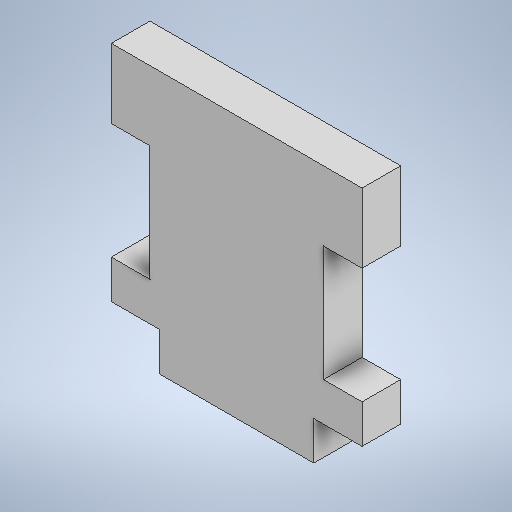
# Autodesk Inventor part: Manija3
Saved by Autodesk Inventor 2025 (Build 290162000, 162)
## iProperties
Created: 2024-11-21
Part Number: Manija3
Material: Generic
Document SubType Name: Sheet Metal
Designer: g.marin
Density: 1 g/cm^3
Sheet Metal Rule: Default
Appearance: Default
Author: g.marin
Autodesk Inventor part; units mm, degrees
ref_plane "YZ Plane" through (0, 0, 0) normal (1, 0, 0) x (0, 1, 0)
ref_plane "XZ Plane" through (0, 0, 0) normal (0, 1, 0) x (-1, 0, 0)
ref_plane "XY Plane" through (0, 0, 0) normal (0, 0, 1) x (1, 0, 0)
sketch "Sketch1" plane through (0, 0, 0) normal (0, 0, 1) x (1, 0, 0)
  line L0 (-16.25, -14.5) -> (16.25, -14.5)
  line L1 (16.25, -14.5) -> (16.25, 14.5)
  line L2 (16.25, 14.5) -> (-16.25, 14.5)
  line L3 (-16.25, 14.5) -> (-16.25, -14.5)
  line L4 (-16.25, -14.5) -> (16.25, 14.5) construction
  line L5 (16.25, -14.5) -> (-16.25, 14.5) construction
  line L6 (-10, -14.5) -> (10, -14.5)
  line L7 (10, -14.5) -> (10, -19.5)
  line L8 (10, -19.5) -> (-10, -19.5)
  line L9 (-10, -19.5) -> (-10, -14.5)
  line L10 (16.25, 5.5) -> (11.25, 5.5)
  line L11 (11.25, 5.5) -> (11.25, -9.5)
  line L12 (11.25, -9.5) -> (16.25, -9.5)
  line L13 (16.25, -9.5) -> (16.25, 5.5)
  line L14 (-16.25, 5.5) -> (-11.25, 5.5)
  line L15 (-11.25, 5.5) -> (-11.25, -9.5)
  line L16 (-11.25, -9.5) -> (-16.25, -9.5)
  line L17 (-16.25, -9.5) -> (-16.25, 5.5)
  point P0 (0, 0)
  point P1 (0, -14.5)
  dimension "d0" = 29
  dimension "d1" = 32.5
  dimension "d2" = 5
  dimension "d3" = 20
  dimension "d4" = 10
  dimension "d5" = 5
  dimension "d6" = 5
  dimension "d7" = 15
  dimension "d8" = 15
  dimension "d9" = 9
  constraints: 36 end point, 8 parallel, 4 horizontal, 4 perpendicular, 4 point on line, 3 midpoint
  measures "d0" distance of L0.end L1.end
  measures "d1" distance of L1.end L2.end
  measures "d2" distance of L6.end L7.end
  measures "d3" distance of L7.end L8.end
  measures "d4" distance from line of point (0, -14.5) L9
  measures "d5" distance of L10.start L10.end
  measures "d6" distance of L14.start L14.end
  measures "d7" distance of L14.end L15.end
  measures "d8" distance of L10.end L11.end
  measures "d9" distance between parallel lines of L14 L2
extrude "Extrusion1" add sketch "Sketch1" along normal blind 5 contours L3 L16 L15 L14 L2 L1 L10 L11 L12 L0 | L0 L7 L8 L9
equation "\"BendRadius\" = Thickness"
equation "\"BendReliefWidth\" = Thickness"
equation "\"BendReliefDepth\" = 0.5 * Thickness"
equation "\"CornerReliefSize\" = 4 * Thickness"
equation "\"MinimumRemnant\" = 2 * Thickness"
equation "\"TransitionRadius\" = BendRadius"
equation "\"JacobiRadiusSize\" = BendRadius"
equation "\"GapSize\" = Thickness"
equation "\"Thickness\" = 3.048"
body "Solid1"
